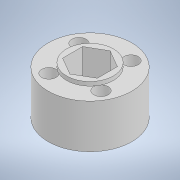
# Autodesk Inventor part: GoBilda Mech Hub 0500 Hex Spacer  inserts
Saved by Autodesk Inventor 2022 (Build 260153000, 153)
## iProperties
Created: 2021-12-21
Part Number: GoBilda Mech Hub 0500 Hex Spacer  inserts
Material: Generic
Document SubType Name: Modeling
Designer: TakeHomePC
Density: 1 g/cm^3
Appearance: Default
Author: TakeHomePC
Autodesk Inventor part; units mm, degrees
ref_plane "YZ Plane" through (0, 0, 0) normal (1, 0, 0) x (0, 1, 0)
ref_plane "XZ Plane" through (0, 0, 0) normal (0, 1, 0) x (-1, 0, 0)
sketch "Sketch1" plane through (0, 0, 0) normal (0, 1, 0) x (-1, 0, 0)
  circle A0 centre (9.798, -5.6569) radius 3.4
  circle A1 centre (0, 0) radius 15.739
  line L0 (0, -7.5575) -> (-6.545, -3.7788)
  line L1 (-6.545, -3.7788) -> (-6.545, 3.7788)
  line L2 (-6.545, 3.7788) -> (0, 7.5575)
  line L3 (0, 7.5575) -> (6.545, 3.7788)
  line L4 (6.545, 3.7788) -> (6.545, -3.7788)
  line L5 (6.545, -3.7788) -> (0, -7.5575)
  circle A2 centre (5.6569, 9.798) radius 3.4
  circle A3 centre (-9.798, 5.6569) radius 3.4
  circle A4 centre (-5.6569, -9.798) radius 3.4
  circle A5 centre (5.6569, 9.798) radius 1.86 projected
  circle A6 centre (0, 0) radius 8.8161
  circle A7 centre (5.6569, 9.798) radius 2.7
  circle A8 centre (-9.798, 5.6569) radius 2.7
  circle A9 centre (-5.6569, -9.798) radius 2.7
  circle A10 centre (9.798, -5.6569) radius 2.7
  point P0 (0, 0)
  dimension "d0" = 31.478
  dimension "d3" = 13.09
  dimension "d4" = 6.8
  dimension "d7" = 360
  dimension "d13" = 5.4
  dimension "d16" = 360
  constraints: 12 end point, 10 centre point, 5 coincident, 31 other
  measures "d0" diameter of A1
  measures "d3" distance between parallel lines of L4 L1
  measures "d4" diameter of A0
  measures "d13" diameter of A7
extrude "Extrusion1" add sketch "Sketch1" along normal blind 16.5 contours A0 A6 A4 A3 A2 | A1
ref_plane "Work Plane1" through (-24.2096, 24.4273, -24.2096) normal (0, 1, 0) x (0.0853, 0, 0.9964)
extrude "Extrusion2" add sketch "Sketch1" along normal blind 1.5 from surface at 16.5 contours A6 A10 A0 | A0 A6 A4 A3 A2 | A6 A10 | A6 A9 A4 | A2 A6 A7 | A6 A9 | A7 A6 | A6 A8 A3 | A6 A8 picked at (7.7135, -3.2903) picked at (7.577, -4.2584) picked at (-3.2903, -7.7135) picked at (5.035, 6.7062) picked at (-4.2584, -7.577) picked at (4.4327, 7.4764) picked at (-6.8562, 4.5301) picked at (-7.577, 4.2584)
extrude "Extrusion4" add sketch "Sketch1" against normal blind 6.5 from surface at 16.5 contours A0 A6 A10 | A6 A10 A0 | A6 A9 A4 | A4 A6 A9 | A6 A7 A2 | A2 A6 A7 | A6 A8 A3 | A3 A6 A8
body "Solid1"
